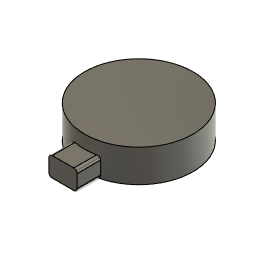
watch-and-dock (Autodesk Fusion 360 archive; units mm, degrees)
design "vibration_motor"
Autodesk Fusion 360 part; units mm, degrees
sketch "Sketch1" plane through (0, 0, 0) normal (0, 1, 0) x (1, 0, 0)
  circle A0 centre (0, 0) radius 5
  line L0 (0, 0) -> (0, -5) construction
  line L1 (0, -5) -> (1.3, -5)
  line L2 (1.3, -5) -> (1.3, -7)
  line L3 (1.3, -7) -> (0, -7)
  line L4 (0, -7) -> (0, -5)
  line L5 (-1.3, -7) -> (0, -7)
  line L6 (-1.3, -5) -> (-1.3, -7)
  line L7 (0, -5) -> (-1.3, -5)
  line L8 (-1.3, -5) -> (-1.3, -4.828)
  line L9 (1.3, -5) -> (1.3, -4.828)
  dimension "d1" = 10
  dimension "d2" = 1.3
  dimension "d3" = 2
  constraint coincident A0.centre L0.start
  constraint coincident A0 L0.end
  constraint vertical L0
  constraint horizontal L1
  constraint vertical L2
  constraint horizontal L3
  constraint vertical L4
  constraint symmetric L0.end L4 L1.start
  constraint symmetric L1.end L4 L6.start
  constraint symmetric L2.end L4 L5.start
  constraint symmetric L3.end L4 L5.end
  constraint coincident A0 L8.end
  constraint perpendicular L7 L8
  constraint coincident A0 L9.end
  constraint perpendicular L1 L9
  measures "d1" diameter of A0
  measures "d2" distance of L0.end L1.end
  measures "d3" distance of L0.end L3.end
extrude "Extrude1" add sketch "Sketch1" along normal blind 3 contours A0
extrude "Extrude2" add sketch "Sketch1" along normal blind 1.8 contours A0 L7 L8 | A0 L1 L9 | L1 L2 L3 L4 | L4 L5 L6 L7
fillet "Fillet1" radius 0.3 4 edges at (-1.3, 1.8, 5.914) (1.3, 1.8, 5.914) (-1.3, 0, 5.914) (1.3, 0, 5.914)
equation "d2 = ( 2.6 / 2 ) * 1 mm"

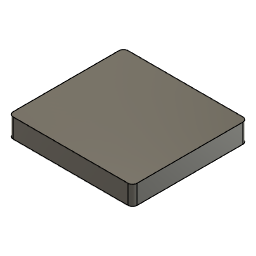
design "battery-200mah"
Autodesk Fusion 360 part; units mm, degrees
sketch "Sketch1" plane through (0, 0, 0) normal (0, 1, 0) x (1, 0, 0)
  line L0 (13.75, -12.75) -> (-13.75, -12.75)
  line L1 (-13.75, -12.75) -> (-13.75, 12.75)
  line L2 (-13.75, 12.75) -> (13.75, 12.75)
  line L3 (13.75, 12.75) -> (13.75, -12.75)
  line L4 (13.75, -12.75) -> (-13.75, 12.75) construction
  line L5 (-13.75, -12.75) -> (13.75, 12.75) construction
  dimension "d1" = 27.5
  dimension "d2" = 25.5
  constraint horizontal L0
  constraint perpendicular L0 L1
  constraint parallel L0 L2
  constraint parallel L1 L3
  constraint coincident L4 origin
  constraint coincident L5 origin
  measures "d1" distance of L1.end L2.end
  measures "d2" distance of L0.end L1.end
extrude "Extrude1" add sketch "Sketch1" along normal blind 4.25
fillet "Fillet1" radius 1 4 edges at (13.75, 2.125, 12.75) (-13.75, 2.125, 12.75) (13.75, 2.125, -12.75) (-13.75, 2.125, -12.75)

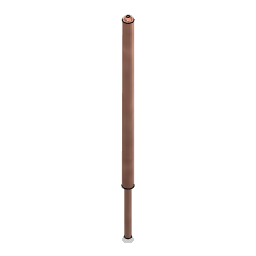
design "pogo-pin"
Autodesk Fusion 360 part; units mm, degrees
sketch "Sketch1" plane through (0, 0, 0) normal (0, 0, 1) x (1, 0, 0)
  line L0 (0, 0) -> (0, -24.4)
  line L1 (0, -24.4) -> (1.4, -24.4)
  line L2 (1.4, -24.4) -> (1.4, 0)
  line L3 (1.4, 0) -> (0, 0)
  line L4 (0.22, -24.4) -> (0.221454, -32.198621)
  line L5 (1.12, -24.4) -> (1.111932, -32.199542)
  line L6 (0.221454, -32.198621) -> (1.111932, -32.199542)
  line L7 (0.666693, -32.199081) -> (1.112394, -31.753381)
  line L8 (0.666693, -32.199081) -> (1.306396, -32.199081) construction
  line L9 (0.666693, -32.199081) -> (0.221371, -31.753759)
  line L10 (0.7, 0) -> (0.666693, -32.199081)
  dimension "d1" = 1.4
  dimension "d5" = 45
  constraint perpendicular L0 L1
  constraint parallel L0 L2
  constraint parallel L1 L3
  constraint vertical L0
  constraint coincident L0.start L3.end
  constraint perpendicular L5 L6
  constraint horizontal L8
  constraint perpendicular L7 L9
  constraint midpoint L3 L10.start
  constraint perpendicular L6 L10
  measures "d1" distance of L0.start L2.end
  measures "d5" angle of L7 L8
revolve "Revolve1" add sketch "Sketch1" angle 360 about axis through (0.7, 0, 0) along (-0.00103441, -0.99999946, 0) contours L1 L2 L3 L10 picked at (1.073333, -8.133333)
revolve "Revolve2" add sketch "Sketch1" angle 360 about axis through (0.7, 0, 0) along (-0.00103441, -0.99999946, 0) contours L1 L5 L7 L10 picked at (0.817949, -29.450821)
fillet "Fillet1" radius 0.5 1 edges at (0.047372, 0.001399, -0.253131)

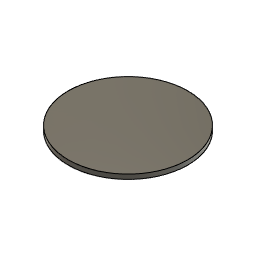
design "glass"
Autodesk Fusion 360 part; units mm, degrees
sketch "Sketch1" plane through (0, 0, 0) normal (0, 1, 0) x (1, 0, 0)
  circle A0 centre (0, 0) radius 19.5
  dimension "d1" = 39
  constraint coincident A0.centre origin
  measures "d1" diameter of A0
extrude "Extrude1" add sketch "Sketch1" along normal blind 1.5

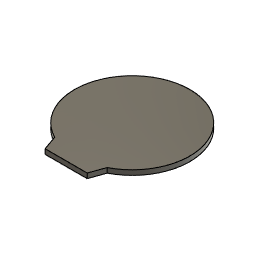
design "display"
Autodesk Fusion 360 part; units mm, degrees
sketch "Sketch1" plane through (0, 0, 0) normal (0, 1, 0) x (1, 0, 0)
  circle A0 centre (0, 0) radius 17.8
  line L0 (-6.5, -20.4) -> (6.5, -20.4)
  line L1 (0, 0) -> (0, -40.8) construction
  line L2 (0, 0) -> (0, 17.8) construction
  line L3 (-8.1, -15.8502) -> (8.1, -15.8502)
  line L4 (6.5, -20.4) -> (8.1, -15.8502)
  line L5 (-8.1, -15.8502) -> (-6.5, -20.4)
  point P0 (0, 17.8)
  dimension "d1" = 35.6
  dimension "d2" = 13
  dimension "d3" = 38.2
  dimension "d4" = 16.2
  constraint coincident A0.centre L1.start
  constraint horizontal L0
  constraint perpendicular L0 L1
  constraint midpoint L0 L1
  constraint coincident A0 P0
  constraint parallel L1 L2
  constraint coincident P0 L2.end
  constraint coincident A0 L3.start
  constraint coincident A0 L3.end
  constraint perpendicular L1 L3
  measures "d1" diameter of A0
  measures "d2" distance of L0.start L0.end
  measures "d3" distance of L0 P0
  measures "d4" distance of L3.start L3.end
extrude "Extrude1" add sketch "Sketch1" along normal blind 1.5
